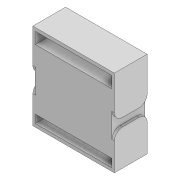
# Autodesk Inventor part: サーボ
Saved by Autodesk Inventor 2020 (Build 240168000, 168)
## iProperties
Created: 2020-04-18
Part Number: サーボ
Material: 一般
Document SubType Name: Modeling
Designer: highs
Density: 1 g/cm^3
Appearance: 既定
Author: highs
Autodesk Inventor part; units mm, degrees
ref_plane "YZ Plane" through (0, 0, 0) normal (1, 0, 0) x (0, 1, 0)
ref_plane "XZ Plane" through (0, 0, 0) normal (0, 1, 0) x (-1, 0, 0)
ref_plane "XY Plane" through (0, 0, 0) normal (0, 0, 1) x (1, 0, 0)
sketch "スケッチ1" plane through (0, 0, 0) normal (0, 0, 1) x (1, 0, 0)
  line L0 (0, 0) -> (50, 0)
  line L1 (50, 0) -> (50, 53)
  line L2 (50, 53) -> (0, 53)
  line L3 (0, 53) -> (0, 0)
  line L4 (1.5, 2) -> (48.5, 2)
  line L5 (48.5, 2) -> (48.5, 7)
  line L6 (48.5, 7) -> (1.5, 7)
  line L7 (1.5, 7) -> (1.5, 2)
  line L8 (1.5, 51) -> (48.5, 51)
  line L9 (48.5, 51) -> (48.5, 44)
  line L10 (48.5, 44) -> (1.5, 44)
  line L11 (1.5, 44) -> (1.5, 51)
  line L12 (0, 27) -> (1.5, 27)
  line L13 (1.5, 27) -> (1.5, 22)
  line L14 (1.5, 22) -> (0, 22)
  line L15 (50, 27) -> (48.5, 27)
  line L16 (48.5, 27) -> (48.5, 22)
  line L17 (48.5, 22) -> (50, 22)
  dimension "d0" = 50
  dimension "d1" = 53
  dimension "d2" = 2
  dimension "d3" = 1.5
  dimension "d4" = 1.5
  dimension "d5" = 5
  dimension "d6" = 2
  dimension "d7" = 7
  dimension "d8" = 5
  dimension "d9" = 17
  constraints: 36 end point, 8 point on line, 7 perpendicular, 6 parallel, 4 horizontal, 3 collinear
  measures "d0" distance of L0.start L0.end
  measures "d1" distance of L2.end L0.start
  measures "d2" distance between parallel lines of L0 L4
  measures "d3" distance between parallel lines of L3 L7
  measures "d4" distance between parallel lines of L1 L5
  measures "d5" distance between parallel lines of L6 L4
  measures "d6" distance between parallel lines of L2 L8
  measures "d7" distance of L10.end L8.start
  measures "d8" distance of L12.end L13.end
  measures "d9" distance between parallel lines of L12 L10
extrude "押し出し1" add sketch "スケッチ1" along normal blind 20.1 contours L3 L14 L13 L12 L2 L1 L15 L16 L17 L0
fillet "フィレット1" radius 5 8 edges at (0.75, 27, 20.1) (0.75, 27, 0) (0.75, 22, 0) (0.75, 22, 20.1) (49.25, 22, 0) (49.25, 22, 20.1) (49.25, 27, 0) (49.25, 27, 20.1)
